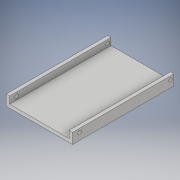
# Autodesk Inventor part: CaseBottom
Saved by Autodesk Inventor 2019 (Build 230136000, 136)
## iProperties
Created: 2019-12-10
Part Number: CaseBottom
Material: 常规
Document SubType Name: Modeling
Designer: cxcyh
Density: 1 g/cm^3
Appearance: 默认
Author: cxcyh
Autodesk Inventor part; units mm, degrees
ref_plane "YZ Plane" through (0, 0, 0) normal (1, 0, 0) x (0, 1, 0)
ref_plane "XZ Plane" through (0, 0, 0) normal (0, 1, 0) x (-1, 0, 0)
ref_plane "XY Plane" through (0, 0, 0) normal (0, 0, 1) x (1, 0, 0)
sketch "草图1" plane through (0, 0, 0) normal (0, 0, 1) x (1, 0, 0)
  line L0 (0, -1.2) -> (0, 7.2) construction
  line L1 (-26.6, 0) -> (26.6, 0) construction
  line L2 (0, 0) -> (-19, 0)
  line L3 (0, 2) -> (-17, 2)
  line L4 (-19, 0) -> (-19, 6)
  line L5 (-19, 6) -> (-17, 6)
  line L6 (-17, 6) -> (-17, 2)
  line L7 (0, 0) -> (19, 0)
  line L8 (0, 2) -> (17, 2)
  line L9 (19, 0) -> (19, 6)
  line L10 (19, 6) -> (17, 6)
  line L11 (17, 6) -> (17, 2)
  dimension "d0" = 19
  dimension "d1" = 17
  dimension "d2" = 2
  dimension "d3" = 6
  constraints: 20 end point, 4 symmetric about line, 2 perpendicular, 2 point on line, 1 horizontal, 1 vertical
  measures "d0" distance of L2.start L2.end
  measures "d1" distance of L3.start L3.end
  measures "d2" distance between parallel lines of L2 L3
  measures "d3" distance of L2.end L4.end
extrude "拉伸1" add sketch "草图1" along normal blind 58
sketch "草图2" plane through (19, 0, 0) normal (1, 0, 0) x (0, 0, -1)
  line L0 (0, 6) -> (0, 0) construction
  line L1 (0, 6) -> (-58, 6) construction
  line L2 (-58, 0) -> (-58, 6) construction
  line L3 (0, 0) -> (-58, 0) construction
  line L4 (0, 2) -> (-58, 2) construction
  line L5 (0, 6) -> (-58, 6) construction
  line L6 (-56, 6) -> (-56, 0) construction
  line L7 (0, 0) -> (-58, 0) construction
  line L8 (-58, 0) -> (-58, 6) construction
  line L9 (-58, 4) -> (0, 4) construction
  circle A0 centre (-54, 4) radius 1
  circle A1 centre (-2, 4) radius 1
  dimension "d6" = 2
  dimension "d7" = 4
  dimension "d8" = 2
  dimension "d9" = 2
  dimension "d10" = 2
  dimension "d11" = 2
  constraints: 6 point on line, 4 end point, 2 centre point, 2 perpendicular
  measures "d6" distance between parallel lines of L2 L6
  measures "d7" diameter of L1 L9
  measures "d8" diameter of A0
  measures "d9" diameter of A1
  measures "d10" distance from line of L6 A0.centre
  measures "d11" distance from line of L0 A1.centre
extrude "拉伸2" cut sketch "草图2" against normal blind 2
mirror "镜像1" about plane through (0, 0, 0) normal (1, 0, 0) of "拉伸2"
